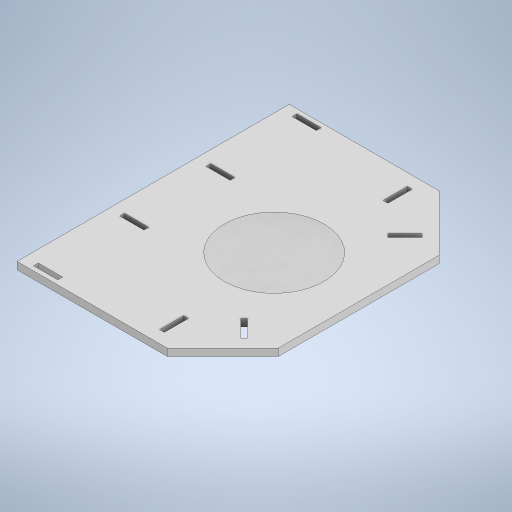
# Autodesk Inventor part: PalmInsert
Saved by Autodesk Inventor 2023 (Build 270158000, 158)
## iProperties
Created: 2023-05-03
Part Number: PalmInsert
Material: Generic
Document SubType Name: Modeling
Designer: 1senadi
Density: 1 g/cm^3
Appearance: Default
Author: 1senadi
Autodesk Inventor part; units mm, degrees
ref_plane "YZ Plane" through (0, 0, 0) normal (1, 0, 0) x (0, 1, 0)
ref_plane "XZ Plane" through (0, 0, 0) normal (0, 1, 0) x (-1, 0, 0)
sketch "Sketch1" plane through (0, 0, 0) normal (0, 1, 0) x (-1, 0, 0)
  line L0 (0, 0) -> (0, -112.4)
  line L1 (0, 0) -> (112.4, 0) construction
  line L2 (0, -112.4) -> (-61.993, -112.4)
  line L3 (0, -112.4) -> (61.993, -112.4) construction
  line L4 (0, 0) -> (-61.993, 0)
  line L5 (0, 0) -> (61.993, 0) construction
  line L6 (-61.993, -112.4) -> (-84.969, -89.424)
  line L7 (-61.993, -112.4) -> (-29.5, -112.4) construction
  line L8 (-61.993, 0) -> (-84.969, -22.976)
  line L9 (-61.993, 0) -> (-29.5, 0) construction
  line L10 (-84.969, -22.976) -> (-84.969, -89.424)
  line L11 (-84.969, -56.2) -> (-89.969, -56.2)
  line L12 (-84.969, -89.424) -> (-89.969, -56.2)
  line L13 (-84.969, -22.976) -> (-89.969, -56.2)
  line L14 (0, -112.4) -> (0, -109.6)
  line L15 (0, -109.6) -> (-5, -109.6)
  line L16 (-5, -109.6) -> (-5, -110.6)
  line L17 (-5, -110.6) -> (-15, -110.6)
  line L18 (-15, -110.6) -> (-15, -108.6)
  line L19 (-15, -108.6) -> (-5, -108.6)
  line L20 (-5, -108.6) -> (-5, -109.6)
  line L21 (-15, -75) -> (-15, -73)
  line L22 (-15, -73) -> (-5, -73)
  line L23 (-5, -75) -> (-15, -75)
  line L24 (-5, -74) -> (-5, -75)
  line L25 (-5, -73) -> (-5, -74)
  line L26 (-15, -39.4) -> (-15, -37.4)
  line L27 (-15, -37.4) -> (-5, -37.4)
  line L28 (-5, -39.4) -> (-15, -39.4)
  line L29 (-5, -38.4) -> (-5, -39.4)
  line L30 (-5, -37.4) -> (-5, -38.4)
  line L31 (-15, -3.8) -> (-15, -1.8)
  line L32 (-15, -1.8) -> (-5, -1.8)
  line L33 (-5, -3.8) -> (-15, -3.8)
  line L34 (-5, -2.8) -> (-5, -3.8)
  line L35 (-5, -1.8) -> (-5, -2.8)
  line L36 (-84.969, -89.424) -> (-77.898, -96.495)
  line L37 (-77.898, -96.495) -> (-74.3624, -92.9595)
  line L38 (-74.3624, -92.9595) -> (-75.0695, -92.2524)
  line L39 (-75.0695, -92.2524) -> (-67.9985, -85.1813)
  line L40 (-67.9985, -85.1813) -> (-66.5842, -86.5956)
  line L41 (-66.5842, -86.5956) -> (-73.6553, -93.6666)
  line L42 (-73.6553, -93.6666) -> (-74.3624, -92.9595)
  line L43 (-74.3624, -19.4405) -> (-75.0695, -20.1476)
  line L44 (-75.0695, -20.1476) -> (-67.9985, -27.2187)
  line L45 (-67.9985, -27.2187) -> (-66.5842, -25.8044)
  line L46 (-66.5842, -25.8044) -> (-73.6553, -18.7334)
  line L47 (-73.6553, -18.7334) -> (-74.3624, -19.4405)
  line L48 (-61.993, -112.4) -> (-54.8, -112.4)
  line L49 (-54.8, -112.4) -> (-54.8, -107.4)
  line L50 (-54.8, -107.4) -> (-55.8, -107.4)
  line L51 (-55.8, -107.4) -> (-55.8, -97.4)
  line L52 (-55.8, -97.4) -> (-53.8, -97.4)
  line L53 (-53.8, -97.4) -> (-53.8, -107.4)
  line L54 (-53.8, -107.4) -> (-54.8, -107.4)
  line L55 (-54.8, -5) -> (-55.8, -5)
  line L56 (-55.8, -5) -> (-55.8, -15)
  line L57 (-55.8, -15) -> (-53.8, -15)
  line L58 (-53.8, -15) -> (-53.8, -5)
  line L59 (-53.8, -5) -> (-54.8, -5)
  dimension "d0" = 112.4
  dimension "d1" = 90
  dimension "d2" = 61.993
  dimension "d3" = 180
  dimension "d4" = 61.993
  dimension "d5" = 180
  dimension "d24" = 32.493
  dimension "d25" = 225
  dimension "d26" = 32.493
  dimension "d27" = 225
  dimension "d28" = 5
  dimension "d29" = 2.8
  dimension "d30" = 5
  dimension "d31" = 1
  dimension "d32" = 10
  dimension "d33" = 2
  dimension "d34" = 10
  dimension "d35" = 90
  dimension "d38" = 35.6
  dimension "d43" = 10
  dimension "d44" = 5
  dimension "d45" = 1
  dimension "d46" = 10
  dimension "d47" = 2
  dimension "d57" = 7.193
  dimension "d58" = 5
  dimension "d59" = 90
  dimension "d60" = 1
  dimension "d61" = 10
  dimension "d62" = 2
  dimension "d63" = 10
  dimension "d64" = 90
  constraints: 120 end point, 15 perpendicular, 10 symmetric about line, 8 horizontal, 5 equal length, 5 point on line, 3 vertical, 1 midpoint, 30 other
  measures "d0" distance of L0.start L0.end
  measures "d1" angle of L0 L1
  measures "d2" distance of L0.end L2.end
  measures "d3" angle of L2 L3
  measures "d4" distance of L0.start L4.end
  measures "d5" angle of L4 L5
  measures "d24" distance of L2.end L6.end
  measures "d26" distance of L4.end L8.end
  measures "d28" distance of L11.start L11.end
  measures "d29" distance of L0.end L14.end
  measures "d30" distance of L14.end L15.end
  measures "d31" distance of L15.end L16.end
  measures "d32" distance of L16.end L17.end
  measures "d33" distance of L17.end L18.end
  measures "d34" distance of L18.end L19.end
  measures "d35" angle of L18 L19
  measures "d38" distance of L17.end L21.start
  measures "d43" distance of L6.end L36.end
  measures "d44" distance of L36.end L37.end
  measures "d45" distance of L37.end L38.end
  measures "d46" distance of L38.end L39.end
  measures "d47" distance of L39.end L40.end
  measures "d57" distance of L2.end L48.end
  measures "d58" distance of L48.end L49.end
  measures "d59" angle of L49 L48
  measures "d60" distance of L49.end L50.end
  measures "d61" distance of L50.end L51.end
  measures "d62" distance of L51.end L52.end
  measures "d63" distance of L52.end L53.end
  measures "d64" angle of L52 L53
extrude "Extrusion1" add sketch "Sketch1" along normal blind 3 contours L0 L2 L6 L10 L8 L4
ref_plane "Work Plane1" through (0, 3, -56.2) normal (0, 0, 1) x (1, 0, 0)
sketch "Sketch4" plane through (0, 3, -56.2) normal (0, 0, 1) x (1, 0, 0)
  line L0 (15, 0) -> (84.969, 0)
  line L1 (84.969, 0) -> (61.993, 0) projected
  line L2 (84.969, 0) -> (49.9845, 0)
  line L3 (61.993, 0) -> (0, 0) projected
  line L4 (49.9845, 0) -> (49.9845, 27.44)
  circle A0 centre (49.9845, 27.44) radius 34.3
  line L5 (49.9845, -6.86) -> (49.9845, 61.74)
  point P0 (0, -3)
  dimension "d53" = 34.9845
  dimension "d54" = 27.44
  dimension "d55" = 68.6
  constraints: 8 end point, 2 point on circle, 1 centre point, 1 coincident, 1 horizontal, 1 perpendicular, 1 point on line, 1 vertical
  measures "d53" distance of L0.end L2.end
  measures "d54" distance of L2.end L4.end
  measures "d55" diameter of A0
revolve "Revolution2" cut sketch "Sketch4" angle 360 about axis through (49.9845, 3, -56.2) along (0, 1, 0) picked at (38.3687, -1.2506) picked at (43.1245, 9.1467) contours L5 A0 L0 | L0 A0 L5 L4
sketch "Sketch6" plane through (0, 3, -56.2) normal (0, 0, 1) x (1, 0, 0)
  line L0 (15, 0) -> (84.969, 0)
  line L1 (84.969, 0) -> (61.993, 0)
  line L2 (84.969, 0) -> (49.9845, 0)
  line L3 (61.993, 0) -> (0, 0)
  line L4 (49.9845, 0) -> (49.9845, 27.44)
  circle A0 centre (49.9845, 27.44) radius 34.3
  line L5 (49.9845, -6.86) -> (49.9845, 61.74)
  circle A1 centre (49.9845, 27.44) radius 37.3
  line L6 (49.9845, -9.86) -> (49.9845, -3)
  line L7 (84.969, -3) -> (61.993, -3) projected
  line L8 (71.5413, -3) -> (28.4277, -3)
  point P0 (0, -3)
  point P1 (0, -3)
  point P2 (65.7926, -3)
  dimension "d70" = 34.9845
  dimension "d71" = 27.44
  dimension "d72" = 68.6
  dimension "d73" = 3
  constraints: 16 end point, 5 point on circle, 3 point on line, 2 centre point, 1 coincident, 1 collinear, 1 horizontal, 1 perpendicular, 1 vertical
  measures "d70" distance of L0.end L2.end
  measures "d71" distance of L2.end L4.end
  measures "d72" diameter of A0
  measures "d73" radial gap between concentric circles of A0 A1
revolve "Revolution4" add sketch "Sketch6" angle 360 about axis through (49.9845, -3.86, -56.2) along (0, 1, 0) contours A0 L7 A1 L6
body "Solid1"
